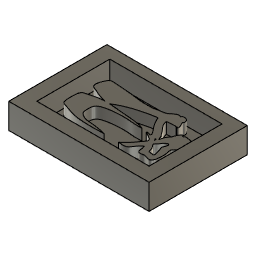
Pointe_Shoe (Autodesk Fusion 360 design; units mm, degrees)
Autodesk Fusion 360 part; units mm, degrees
sketch "Sketch1" plane through (0, 0, 0) normal (0, 0, 1) x (1, 0, 0)
  spline S0 degree 5 poles (-11.1843, -2.2894) (-11.167, -2.3096) (-11.1327, -2.3492) (-11.0825, -2.4064) (-11.0179, -2.4782) (-10.9409, -2.5607) (-10.8672, -2.6362) (-10.7955, -2.7054) (-10.7238, -2.7696) (-10.6489, -2.8307) (-10.5674, -2.891) (-10.4761, -2.9527) (-10.3728, -3.0176) (-10.2574, -3.0865) (-10.1318, -3.1589) (-9.9991, -3.2339) (-9.8634, -3.3097) (-9.7286, -3.3844) (-9.5981, -3.4561) (-9.4738, -3.5232) (-9.3565, -3.5843) (-9.2459, -3.6385) (-9.1414, -3.6849) (-9.0421, -3.7231) (-8.9473, -3.7527) (-8.8567, -3.7736) (-8.7873, -3.7834) (-8.7369, -3.7869) (-8.7041, -3.7874) (-8.6879, -3.7873) knots 0 0 0 0 0 0 0.04 0.08 0.12 0.16 0.2 0.24 0.28 0.32 0.36 0.4 0.44 0.48 0.52 0.56 0.6 0.64 0.68 0.72 0.76 0.8 0.84 0.88 0.92 0.96 1 1 1 1 1 1
  spline S1 degree 5 poles (4.0148, 3.4427) (3.8783, 3.4353) (3.6103, 3.4218) (3.2238, 3.4053) (2.7393, 3.3909) (2.1844, 3.3854) (1.6785, 3.3922) (1.218, 3.4101) (0.7966, 3.438) (0.405, 3.4734) (0.0299, 3.5135) (-0.3435, 3.5544) (-0.7292, 3.5927) (-1.138, 3.6252) (-1.5741, 3.6497) (-2.0345, 3.6652) (-2.512, 3.6716) (-2.9969, 3.6695) (-3.4802, 3.6596) (-3.9557, 3.6428) (-4.4224, 3.6197) (-4.8836, 3.5905) (-5.3447, 3.5552) (-5.8119, 3.5134) (-6.2904, 3.4642) (-6.7826, 3.4063) (-7.2875, 3.3381) (-7.8013, 3.2575) (-8.3174, 3.1622) (-8.8273, 3.0498) (-9.3207, 2.9176) (-9.7857, 2.763) (-10.21, 2.5834) (-10.5824, 2.3753) (-10.8943, 2.1343) (-11.1409, 1.8548) (-11.3232, 1.5288) (-11.4473, 1.1483) (-11.522, 0.7091) (-11.5571, 0.2147) (-11.5606, -0.3207) (-11.537, -0.8664) (-11.4865, -1.3808) (-11.4055, -1.8231) (-11.31, -2.0996) (-11.2166, -2.2572) (-11.1425, -2.3444) (-11.1014, -2.3849) (-11.0994, -2.3868) knots 0 0 0 0 0 0 0.014286 0.028571 0.042857 0.057143 0.071429 0.085714 0.1 0.114286 0.128571 0.142857 0.157143 0.171429 0.185714 0.2 0.214286 0.228571 0.242857 0.257143 0.271429 0.285714 0.3 0.314286 0.328571 0.342857 0.357143 0.371429 0.385714 0.4 0.414286 0.428571 0.442857 0.457143 0.471429 0.485714 0.5 0.514286 0.528571 0.542857 0.557143 0.571429 0.585714 0.6 0.614286 0.615002 0.615002 0.615002 0.615002 0.615002 0.615002
  line L0 (-12.4584, -1.0588) -> (-9.7404, -3.7149)
  spline S2 degree 5 poles (-8.6879, -3.7873) (-8.6225, -3.8062) (-8.4825, -3.8421) (-8.2453, -3.8901) (-7.8792, -3.9433) (-7.3672, -3.9951) (-6.8379, -4.0368) (-6.3286, -4.0733) (-5.87, -4.1091) (-5.4766, -4.1473) (-5.1428, -4.1887) (-4.851, -4.2334) (-4.5778, -4.2808) (-4.301, -4.3301) (-4.0067, -4.3817) (-3.6897, -4.4364) (-3.3499, -4.4957) (-2.9908, -4.5607) (-2.6162, -4.6327) (-2.2288, -4.7122) (-1.8301, -4.7996) (-1.503, -4.8758) (-1.2532, -4.9365) (-1.0847, -4.9786) (-1, -5) knots 0 0 0 0 0 0 0.05 0.1 0.15 0.2 0.25 0.3 0.35 0.4 0.45 0.5 0.55 0.6 0.65 0.7 0.75 0.8 0.85 0.9 0.95 1 1 1 1 1 1
  line L1 (-9.2399, -3.6277) -> (-8.1358, -3.9468)
  spline S3 degree 5 poles (9.6142, 10.026) (9.6212, 10.039) (9.6388, 10.0609) (9.6761, 10.0818) (9.7474, 10.0856) (9.8704, 10.0531) (10.0203, 9.9927) (10.1831, 9.923) (10.3362, 9.8739) (10.4544, 9.8782) (10.5157, 9.9641) (10.5061, 10.1473) (10.4263, 10.4231) (10.2881, 10.7708) (10.1115, 11.1587) (9.9211, 11.5502) (9.7427, 11.9083) (9.5999, 12.2013) (9.5109, 12.4077) (9.4852, 12.5219) (9.5196, 12.5594) (9.596, 12.5616) (9.6883, 12.5778) (9.7702, 12.6495) (9.8232, 12.7907) (9.8366, 12.9926) (9.8066, 13.2316) (9.7349, 13.4774) (9.6278, 13.7) (9.4957, 13.8772) (9.3512, 14.0031) (9.2077, 14.0835) (9.076, 14.1314) (8.9623, 14.1621) (8.8658, 14.1892) (8.7751, 14.2189) (8.673, 14.2508) (8.5433, 14.2803) (8.3765, 14.3002) (8.1778, 14.3029) (7.9662, 14.282) (7.7663, 14.2336) (7.6026, 14.1578) (7.4921, 14.06) (7.4383, 13.9526) (7.4236, 13.8563) (7.4193, 13.7932) (7.3957, 13.779) (7.3349, 13.8141) (7.2335, 13.883) (7.0966, 13.9633) (6.9346, 14.0313) (6.7579, 14.071) (6.5743, 14.0766) (6.3902, 14.0492) (6.2103, 13.9947) (6.0374, 13.9214) (5.8732, 13.8375) (5.7178, 13.7485) (5.5707, 13.6572) (5.4304, 13.5647) (5.2956, 13.4708) (5.1651, 13.3751) (5.0383, 13.2773) (4.9157, 13.1779) (4.7981, 13.0778) (4.6859, 12.9784) (4.5792, 12.8811) (4.4765, 12.7872) (4.375, 12.6976) (4.2709, 12.6132) (4.1603, 12.5345) (4.0392, 12.4619) (3.9047, 12.3958) (3.7548, 12.3363) (3.5884, 12.2835) (3.4417, 12.2467) (3.3239, 12.2222) (3.2419, 12.2072) (3.2, 12.2) knots 0 0 0 0 0 0 0.01333333 0.02666667 0.04 0.05333333 0.06666667 0.08 0.09333333 0.10666667 0.12 0.13333333 0.14666667 0.16 0.17333333 0.18666667 0.2 0.21333333 0.22666667 0.24 0.25333333 0.26666667 0.28 0.29333333 0.30666667 0.32 0.33333333 0.34666667 0.36 0.37333333 0.38666667 0.4 0.41333333 0.42666667 0.44 0.45333333 0.46666667 0.48 0.49333333 0.50666667 0.52 0.53333333 0.54666667 0.56 0.57333333 0.58666667 0.6 0.61333333 0.62666667 0.64 0.65333333 0.66666667 0.68 0.69333333 0.70666667 0.72 0.73333333 0.74666667 0.76 0.77333333 0.78666667 0.8 0.81333333 0.82666667 0.84 0.85333333 0.86666667 0.88 0.89333333 0.90666667 0.92 0.93333333 0.94666667 0.96 0.97333333 0.98666667 1 1 1 1 1 1
  spline S4 degree 5 poles (2, 12) (2.048, 12.008) (2.144, 12.024) (2.288, 12.048) (2.48, 12.08) (2.72, 12.12) (2.912, 12.152) (3.056, 12.176) (3.152, 12.192) (3.2, 12.2) knots 0 0 0 0 0 0 0.2 0.4 0.6 0.8 1 1 1 1 1 1
  spline S5 degree 5 poles (2, 12) (1.9505, 11.9948) (1.8529, 11.984) (1.7107, 11.9662) (1.5296, 11.9392) (1.3172, 11.9004) (1.118, 11.8567) (0.9303, 11.8092) (0.7508, 11.7593) (0.5745, 11.7095) (0.3951, 11.6629) (0.2065, 11.6225) (0.0045, 11.5906) (-0.2127, 11.5683) (-0.4425, 11.5551) (-0.6794, 11.549) (-0.9162, 11.5474) (-1.1452, 11.5472) (-1.3596, 11.5458) (-1.5546, 11.5413) (-1.7278, 11.5326) (-1.8481, 11.5219) (-1.9281, 11.5118) (-1.9768, 11.5041) (-2, 11.5) knots 0 0 0 0 0 0 0.05 0.1 0.15 0.2 0.25 0.3 0.35 0.4 0.45 0.5 0.55 0.6 0.65 0.7 0.75 0.8 0.85 0.9 0.95 1 1 1 1 1 1
  spline S6 degree 5 poles (-3.9672, 11.5464) (-4.025, 11.5517) (-4.1405, 11.5622) (-4.3137, 11.5779) (-4.5447, 11.599) (-4.8335, 11.6253) (-5.0645, 11.6463) (-5.2378, 11.662) (-5.3533, 11.6726) (-5.411, 11.6778) knots 0 0 0 0 0 0 0.2 0.4 0.6 0.8 1 1 1 1 1 1
  spline S7 degree 5 poles (-2, 11.5) (-2.1116, 11.5015) (-2.329, 11.5045) (-2.6376, 11.5094) (-3.0142, 11.5163) (-3.429, 11.5261) (-3.7945, 11.5378) (-4.1243, 11.5528) (-4.4418, 11.5739) (-4.7789, 11.6044) (-5.1685, 11.6476) (-5.6391, 11.7054) (-6.2075, 11.7775) (-6.8769, 11.8614) (-7.64, 11.9528) (-8.4809, 12.0469) (-9.3773, 12.1388) (-10.3028, 12.224) (-11.229, 12.2999) (-12.1273, 12.3657) (-12.9715, 12.4238) (-13.7395, 12.4772) (-14.4143, 12.5278) (-14.9866, 12.5734) (-15.4556, 12.6057) (-15.8312, 12.6081) (-16.1363, 12.5523) (-16.4047, 12.4001) (-16.6687, 12.1177) (-16.9492, 11.6855) (-17.242, 11.1144) (-17.518, 10.4443) (-17.7367, 9.7313) (-17.8546, 9.038) (-17.837, 8.4217) (-17.6665, 7.9249) (-17.3563, 7.5626) (-16.9522, 7.3178) (-16.5127, 7.1553) (-16.0928, 7.0332) (-15.7276, 6.9134) (-15.4118, 6.7751) (-15.1095, 6.6135) (-14.7757, 6.4337) (-14.3731, 6.2459) (-13.8942, 6.0591) (-13.3587, 5.8807) (-12.8024, 5.7165) (-12.2684, 5.5708) (-11.7983, 5.4466) (-11.4216, 5.346) (-11.206, 5.2849) (-11.0947, 5.2502) (-11.0428, 5.232) (-11.0225, 5.2241) knots 0 0 0 0 0 0 0.02 0.04 0.06 0.08 0.1 0.12 0.14 0.16 0.18 0.2 0.22 0.24 0.26 0.28 0.3 0.32 0.34 0.36 0.38 0.4 0.42 0.44 0.46 0.48 0.5 0.52 0.54 0.56 0.58 0.6 0.62 0.64 0.66 0.68 0.7 0.72 0.74 0.76 0.78 0.8 0.82 0.84 0.86 0.88 0.9 0.92 0.94 0.96 0.98 1 1 1 1 1 1
  spline S8 degree 5 poles (4.0148, 3.4427) (3.8887, 3.4949) (3.6281, 3.596) (3.2125, 3.7383) (2.609, 3.9092) (1.7731, 4.092) (0.8587, 4.2454) (-0.1284, 4.3727) (-1.1777, 4.479) (-2.2738, 4.5724) (-3.3981, 4.6617) (-4.5314, 4.7545) (-5.656, 4.8558) (-6.7583, 4.9655) (-7.6991, 5.0635) (-8.4088, 5.1313) (-8.9025, 5.1705) (-9.1876, 5.1893) (-9.2671, 5.1943) knots 0 0 0 0 0 0 0.02 0.04 0.06 0.08 0.1 0.12 0.14 0.16 0.18 0.2 0.22 0.24 0.26 0.267756 0.267756 0.267756 0.267756 0.267756 0.267756
  line L2 (-7.9272, 5.1108) -> (-10.607, 5.2777)
  spline S9 degree 5 poles (-11.0225, 5.2241) (-11.1998, 5.2175) (-11.5778, 5.1974) (-12.1554, 5.1467) (-12.9304, 5.0358) (-13.8902, 4.8332) (-14.8317, 4.5921) (-15.6961, 4.3582) (-16.4481, 4.1622) (-17.0602, 4.0074) (-17.5215, 3.8527) (-17.8464, 3.5928) (-18.063, 3.1132) (-18.2006, 2.3488) (-18.276, 1.3464) (-18.2953, 0.2279) (-18.2564, -0.8529) (-18.1506, -1.7534) (-17.9656, -2.3797) (-17.6869, -2.7412) (-17.3014, -2.936) (-16.8022, -3.0842) (-16.194, -3.2658) (-15.4925, -3.501) (-14.7183, -3.7779) (-13.8925, -4.065) (-13.0313, -4.3318) (-12.1419, -4.5616) (-11.2253, -4.7474) (-10.2782, -4.8895) (-9.2946, -4.9925) (-8.2679, -5.063) (-7.1931, -5.1062) (-6.0667, -5.1257) (-4.8865, -5.1242) (-3.6513, -5.103) (-2.6186, -5.0711) (-1.819, -5.0388) (-1.2749, -5.0135) (-1, -5) knots 0.302378 0.302378 0.302378 0.302378 0.302378 0.302378 0.32 0.34 0.36 0.38 0.4 0.42 0.44 0.46 0.48 0.5 0.52 0.54 0.56 0.58 0.6 0.62 0.64 0.66 0.68 0.7 0.72 0.74 0.76 0.78 0.8 0.82 0.84 0.86 0.88 0.9 0.92 0.94 0.96 0.98 1 1 1 1 1 1
  line L3 (-8.0902, 5.3338) -> (-13.9548, 5.1144)
  spline S10 degree 5 poles (6, 3) (6.1626, 2.9146) (6.4768, 2.7481) (6.9154, 2.5109) (7.4345, 2.2202) (7.9733, 1.8987) (8.402, 1.6171) (8.7212, 1.3715) (8.9327, 1.1545) (9.0401, 0.9549) (9.0495, 0.7564) (8.9696, 0.5377) (8.8115, 0.2784) (8.5885, -0.0363) (8.3157, -0.41) (8.0099, -0.831) (7.688, -1.2777) (7.3658, -1.7242) (7.0565, -2.1441) (6.7694, -2.5169) (6.5089, -2.8312) (6.2721, -3.0922) (6.0509, -3.3176) (5.8351, -3.5296) (5.6157, -3.7489) (5.3871, -3.9868) (5.1508, -4.2387) (4.9136, -4.4882) (4.6843, -4.7133) (4.4724, -4.8915) (4.2847, -5.0059) (4.1566, -5.0404) (4.0733, -5.0331) (4.0235, -5.0135) (4, -5) knots 0 0 0 0 0 0 0.033333 0.066667 0.1 0.133333 0.166667 0.2 0.233333 0.266667 0.3 0.333333 0.366667 0.4 0.433333 0.466667 0.5 0.533333 0.566667 0.6 0.633333 0.666667 0.7 0.733333 0.766667 0.8 0.833333 0.866667 0.9 0.933333 0.966667 1 1 1 1 1 1
  spline S11 degree 5 poles (4, -5) (4.139, -5.0271) (4.4102, -5.0769) (4.7968, -5.1386) (5.272, -5.1946) (5.798, -5.2201) (6.2563, -5.2007) (6.6483, -5.1361) (6.978, -5.0267) (7.2527, -4.8739) (7.4841, -4.6807) (7.6865, -4.4515) (7.8744, -4.1919) (8.0607, -3.9092) (8.2538, -3.6117) (8.4567, -3.3092) (8.6688, -3.0113) (8.8874, -2.7274) (9.1089, -2.4653) (9.3301, -2.2305) (9.5496, -2.0257) (9.723, -1.8869) (9.8518, -1.7968) (9.9371, -1.743) (9.9795, -1.7176) knots 0 0 0 0 0 0 0.05 0.1 0.15 0.2 0.25 0.3 0.35 0.4 0.45 0.5 0.55 0.6 0.65 0.7 0.75 0.8 0.85 0.9 0.95 1 1 1 1 1 1
  spline S12 degree 5 poles (9.9795, -1.7176) (10.007, -1.7591) (10.0593, -1.8449) (10.1302, -1.9818) (10.2093, -2.1805) (10.2836, -2.4553) (10.3358, -2.7536) (10.3713, -3.0703) (10.399, -3.3962) (10.4323, -3.718) (10.4889, -4.0175) (10.5867, -4.2761) (10.7397, -4.4772) (10.9544, -4.6101) (11.2261, -4.6727) (11.5348, -4.6753) (11.8525, -4.6359) (12.1494, -4.5765) (12.4017, -4.5184) (12.5975, -4.4787) (12.7461, -4.4649) (12.8756, -4.4749) (13.0176, -4.5023) (13.1945, -4.5414) (13.4082, -4.5905) (13.6485, -4.6499) (13.8992, -4.7195) (14.1443, -4.7974) (14.3753, -4.8773) (14.5923, -4.9485) (14.7994, -4.998) (15.0021, -5.012) (15.2039, -4.9775) (15.4032, -4.8836) (15.5949, -4.7227) (15.7723, -4.4905) (15.9284, -4.1875) (16.0579, -3.819) (16.1587, -3.3962) (16.2311, -2.9342) (16.2775, -2.4506) (16.3013, -1.964) (16.3068, -1.4918) (16.2982, -1.0495) (16.2791, -0.648) (16.2518, -0.2932) (16.2169, 0.0171) (16.1733, 0.2915) (16.1205, 0.5417) (16.0594, 0.7799) (15.9944, 1.0157) (15.9348, 1.2533) (15.8957, 1.4886) (15.8941, 1.7136) (15.944, 1.9204) (16.0533, 2.1048) (16.2178, 2.2714) (16.4225, 2.433) (16.6455, 2.6061) (16.8629, 2.8077) (17.0521, 3.051) (17.1965, 3.3418) (17.2881, 3.676) (17.3263, 4.0427) (17.3163, 4.427) (17.2675, 4.8126) (17.193, 5.1843) (17.1076, 5.5308) (17.0268, 5.8479) (16.9652, 6.1388) (16.9341, 6.4109) (16.9396, 6.6728) (16.9799, 6.9313) (17.0439, 7.189) (17.1076, 7.4404) (17.1394, 7.6743) (17.1081, 7.8784) (16.9897, 8.0428) (16.7757, 8.1648) (16.4779, 8.2513) (16.1214, 8.3138) (15.7388, 8.3653) (15.3647, 8.4156) (15.0294, 8.4679) (14.7536, 8.5145) (14.5417, 8.5325) (14.3854, 8.4955) (14.27, 8.3901) (14.1788, 8.229) (14.0986, 8.0682) (14.0201, 7.9758) (13.9378, 8.0005) (13.8508, 8.1322) (13.7599, 8.3177) (13.6644, 8.489) (13.5584, 8.5919) (13.4318, 8.5991) (13.2768, 8.5023) (13.095, 8.3094) (12.8978, 8.0404) (12.7013, 7.7226) (12.5229, 7.3861) (12.3767, 7.0599) (12.2701, 6.767) (12.1992, 6.5201) (12.1472, 6.3185) (12.092, 6.1524) (12.0125, 6.005) (11.8946, 5.8557) (11.7381, 5.6832) (11.5528, 5.4682) (11.3546, 5.1966) (11.1613, 4.863) (10.9895, 4.4738) (10.8497, 4.0497) (10.743, 3.6303) (10.6626, 3.2653) (10.5976, 3.0042) (10.5356, 2.8859) (10.4661, 2.9299) (10.3835, 3.1238) (10.289, 3.4209) (10.1873, 3.7583) (10.0847, 4.0718) (9.9859, 4.3119) (9.8927, 4.4585) (9.8003, 4.5387) (9.7017, 4.6029) (9.5911, 4.6998) (9.4688, 4.8471) (9.3399, 5.0359) (9.2108, 5.2442) (9.0872, 5.4472) (8.9707, 5.6301) (8.8586, 5.7918) (8.7459, 5.9382) (8.627, 6.0792) (8.4975, 6.2238) (8.3551, 6.3771) (8.1994, 6.542) (8.0316, 6.7198) (7.8541, 6.9107) (7.6704, 7.1148) (7.4844, 7.332) (7.3006, 7.5622) (7.1234, 7.8053) (6.9569, 8.061) (6.8042, 8.3293) (6.6678, 8.61) (6.5492, 8.903) (6.4492, 9.2082) (6.3846, 9.4622) (6.3448, 9.6582) (6.3221, 9.7914) (6.3117, 9.8585) knots 0 0 0 0 0 0 0.00666667 0.01333333 0.02 0.02666667 0.03333333 0.04 0.04666667 0.05333333 0.06 0.06666667 0.07333333 0.08 0.08666667 0.09333333 0.1 0.10666667 0.11333333 0.12 0.12666667 0.13333333 0.14 0.14666667 0.15333333 0.16 0.16666667 0.17333333 0.18 0.18666667 0.19333333 0.2 0.20666667 0.21333333 0.22 0.22666667 0.23333333 0.24 0.24666667 0.25333333 0.26 0.26666667 0.27333333 0.28 0.28666667 0.29333333 0.3 0.30666667 0.31333333 0.32 0.32666667 0.33333333 0.34 0.34666667 0.35333333 0.36 0.36666667 0.37333333 0.38 0.38666667 0.39333333 0.4 0.40666667 0.41333333 0.42 0.42666667 0.43333333 0.44 0.44666667 0.45333333 0.46 0.46666667 0.47333333 0.48 0.48666667 0.49333333 0.5 0.50666667 0.51333333 0.52 0.52666667 0.53333333 0.54 0.54666667 0.55333333 0.56 0.56666667 0.57333333 0.58 0.58666667 0.59333333 0.6 0.60666667 0.61333333 0.62 0.62666667 0.63333333 0.64 0.64666667 0.65333333 0.66 0.66666667 0.67333333 0.68 0.68666667 0.69333333 0.7 0.70666667 0.71333333 0.72 0.72666667 0.73333333 0.74 0.74666667 0.75333333 0.76 0.76666667 0.77333333 0.78 0.78666667 0.79333333 0.8 0.80666667 0.81333333 0.82 0.82666667 0.83333333 0.84 0.84666667 0.85333333 0.86 0.86666667 0.87333333 0.88 0.88666667 0.89333333 0.9 0.90666667 0.91333333 0.92 0.92666667 0.93333333 0.94 0.94666667 0.95333333 0.96 0.96666667 0.97333333 0.98 0.98666667 0.99333333 1 1 1 1 1 1
  spline S13 degree 5 poles (3.647, 9.5084) (3.6997, 9.4048) (3.8036, 9.2012) (3.9549, 8.9067) (4.1475, 8.5361) (4.3731, 8.1092) (4.5851, 7.7174) (4.7864, 7.3576) (4.9821, 7.0242) (5.18, 6.7081) (5.3915, 6.3963) (5.6285, 6.0741) (5.9003, 5.7283) (6.2099, 5.3505) (6.5513, 4.9396) (6.9054, 4.5052) (7.2378, 4.0701) (7.509, 3.6639) (7.682, 3.3177) (7.7318, 3.0586) (7.6526, 2.9042) (7.4715, 2.8572) (7.2359, 2.9006) (6.9925, 3.0029) (6.7534, 3.104) (6.5085, 3.152) (6.3085, 3.1318) (6.1553, 3.08) (6.052, 3.0294) (6, 3) knots 0 0 0 0 0 0 0.04 0.08 0.12 0.16 0.2 0.24 0.28 0.32 0.36 0.4 0.44 0.48 0.52 0.56 0.6 0.64 0.68 0.72 0.76 0.8 0.84 0.88 0.92 0.96 1 1 1 1 1 1
  spline S14 degree 5 poles (12.5, -2.5) (12.5233, -2.5221) (12.5764, -2.5576) (12.6791, -2.5879) (12.8741, -2.6023) (13.2276, -2.6385) (13.6618, -2.7155) (14.1182, -2.8167) (14.4335, -2.7691) (14.5235, -2.469) (14.4332, -1.9661) (14.2519, -1.3631) (14.0732, -0.7831) (13.957, -0.3209) (13.8354, 0.0299) (13.6935, 0.3071) (13.5613, 0.5552) (13.482, 0.8198) (13.4934, 1.1344) (13.5993, 1.5074) (13.7634, 1.9199) (13.93, 2.3368) (14.0378, 2.7149) (14.0372, 3.0127) (13.9044, 3.1987) (13.6595, 3.261) (13.349, 3.2039) (13.0268, 3.0432) (12.7361, 2.8022) (12.4889, 2.5074) (12.2749, 2.1861) (12.0723, 1.8633) (11.8595, 1.5598) (11.6247, 1.2896) (11.3796, 1.0566) (11.1608, 0.8544) (11.012, 0.6697) (10.9709, 0.4852) (11.0531, 0.2823) (11.2398, 0.0446) (11.4913, -0.2398) (11.7586, -0.5755) (11.9959, -0.9563) (12.1719, -1.3635) (12.2836, -1.7613) (12.3497, -2.1081) (12.3924, -2.3162) (12.4366, -2.4249) (12.4767, -2.4779) (12.5, -2.5) knots 0 0 0 0 0 0 0.022222 0.044444 0.066667 0.088889 0.111111 0.133333 0.155556 0.177778 0.2 0.222222 0.244444 0.266667 0.288889 0.311111 0.333333 0.355556 0.377778 0.4 0.422222 0.444444 0.466667 0.488889 0.511111 0.533333 0.555556 0.577778 0.6 0.622222 0.644444 0.666667 0.688889 0.711111 0.733333 0.755556 0.777778 0.8 0.822222 0.844444 0.866667 0.888889 0.911111 0.933333 0.955556 0.977778 1 1 1 1 1 1
  spline S15 degree 5 poles (-9.2671, 5.1943) (-9.0708, 5.3122) (-8.6752, 5.5444) (-8.0731, 5.8813) (-7.253, 6.3078) (-6.1987, 6.8025) (-5.1159, 7.2582) (-4.0063, 7.6744) (-2.8735, 8.051) (-1.7233, 8.3885) (-0.5646, 8.6883) (0.5918, 8.9527) (1.6767, 9.1722) (2.5141, 9.3239) (3.1134, 9.4242) (3.4878, 9.4837) (3.647, 9.5084) knots 0 0 0 0 0 0 0.05 0.1 0.15 0.2 0.25 0.3 0.35 0.4 0.45 0.5 0.55 0.587521 0.587521 0.587521 0.587521 0.587521 0.587521
  line L4 (2.3392, 9.3051) -> (4.9547, 9.7118)
  spline S16 degree 5 poles (6.3117, 9.8585) (6.407, 9.8686) (6.6776, 9.8964) (7.1098, 9.9374) (7.6776, 9.9835) (8.3399, 10.0226) (8.9853, 10.0411) (9.4334, 10.0366) (9.7314, 10.0225) (9.9133, 10.0083) (10, 10) knots 0.72327 0.72327 0.72327 0.72327 0.72327 0.72327 0.75 0.8 0.85 0.9 0.95 1 1 1 1 1 1
  line L5 (5.8982, 9.8149) -> (6.7253, 9.9021)
  line L6 (7.9699, 2.6099) -> (6.0301, 3.3901)
  line L7 (14.2611, -1.4231) -> (13.7389, 0.4231)
  line L8 (13.4227, -2.7289) -> (14.6526, -2.8257)
  line L9 (14.2611, -1.4231) -> (14.5, -2.8)
  line L10 (10, 2.5) -> (9.6005, 2.5993)
  line L11 (9.6005, 2.5993) -> (10, 2)
  line L12 (10, 2) -> (10, 2.5)
  point P0 (-0.1076, 4.3633)
  point P1 (-7.056, 4.9968)
  point P2 (-13.056, 4.9968)
  point P3 (-17.056, 3.9968)
  point P4 (-18.056, 2.9968)
  point P5 (-18.056, -2.0032)
  point P6 (-17.056, -3.0032)
  point P7 (-14.056, -4.0032)
  point P8 (-9.056, -5.0032)
  point P9 (0.7673, 3.4427)
  point P10 (-1.0205, 3.6145)
  point P11 (-3.5165, 3.6568)
  point P12 (-6.0548, 3.4876)
  point P13 (-9, 3)
  point P14 (-11, 2)
  point P15 (-11.5545, 0)
  point P16 (-11.1843, -2.2894)
  point P17 (-6, -4.1)
  point P18 (-4.4895, -4.2966)
  point P19 (-3.0511, -4.5505)
  point P20 (-10.8, -2.7)
  point P21 (-10.4, -3)
  point P22 (-9.7, -3.4)
  point P23 (-9.1, -3.7)
  point P24 (-3, 8)
  point P25 (8, 10)
  point P26 (10.5, 10)
  point P27 (9.5, 12.5)
  point P28 (9.7, 12.6)
  point P29 (9.6142, 13.701)
  point P30 (8.9417, 14.1681)
  point P31 (8.4633, 14.2877)
  point P32 (7.5, 14.05)
  point P33 (7.4041, 13.7923)
  point P34 (7, 14)
  point P35 (6, 13.9)
  point P36 (5.2, 13.4)
  point P37 (4.6, 12.9)
  point P38 (4.1, 12.5)
  point P39 (0.9, 11.8)
  point P40 (-0.0122, 11.5913)
  point P41 (-1.2257, 11.5464)
  point P42 (-11.2999, 12.3035)
  point P43 (-15.7, 12.6)
  point P44 (-16.8, 11.9)
  point P45 (-17.7, 8.1)
  point P46 (-16, 7)
  point P47 (-14.6566, 6.3821)
  point P48 (-12, 5.5)
  point P49 (9, 1)
  point P50 (8.6094, -0.0043)
  point P51 (6.6911, -2.6076)
  point P52 (5.595, -3.7723)
  point P53 (4.5331, -4.8342)
  point P54 (7, -5)
  point P55 (8, -4)
  point P56 (9.0204, -2.5734)
  point P57 (10.3906, -3.2927)
  point P58 (10.9729, -4.5944)
  point P59 (12.5, -4.5)
  point P60 (13, -4.5)
  point P61 (13.999, -4.7524)
  point P62 (15, -5)
  point P63 (15.9154, -4.1861)
  point P64 (16.2668, -0.5069)
  point P65 (16, 1)
  point P66 (16, 2)
  point P67 (17, 3)
  point P68 (17.1414, 5.3901)
  point P69 (17, 7)
  point P70 (17, 8)
  point P71 (15.0046, 8.4726)
  point P72 (14.269, 8.3675)
  point P73 (14, 8)
  point P74 (13.7086, 8.4025)
  point P75 (13.3583, 8.5427)
  point P76 (12.3074, 6.8613)
  point P77 (12, 6)
  point P78 (10.9763, 4.4093)
  point P79 (10.4859, 2.9381)
  point P80 (9.9795, 4.3042)
  point P81 (9.6756, 4.6297)
  point P82 (9.1529, 5.3391)
  point P83 (8.6675, 6.0298)
  point P84 (8.0141, 6.7392)
  point P85 (7, 8)
  point P86 (5, 7)
  point P87 (6.5, 5)
  point P88 (7.6836, 3.0081)
  point P89 (7, 3)
  point P90 (14.0376, -2.7773)
  point P91 (14, -0.5)
  point P92 (13.5, 1)
  point P93 (14, 3)
  point P94 (13, 3)
  point P95 (11.7119, 1.3968)
  point P96 (11, 0.5)
  point P97 (12, -1)
  constraint coincident P16 S0.start
  constraint coincident S0.end S2.start
  constraint coincident S0 S1.end
  constraint midpoint S1.end L0
  constraint midpoint S0.end L1
  constraint coincident S3.start S16
  constraint midpoint S8.end L2
  constraint midpoint S7.end L3
  constraint coincident S13.start S15.end
  constraint midpoint S13.start L4
  constraint midpoint S12.end L5
  constraint midpoint P89 L6
  constraint midpoint P91 L7
  constraint midpoint P90 L8
  constraint coincident L7.start L9.start
extrude "Extrude1" add sketch "Sketch1" along normal blind 2 contours S0 S1 S2 S8 L2 S9 L3 | L2 L3 S15 | S3 S4 S5 S7 L3 S10 S11 S12 S13 S15 S16 L5 makes body 1
sketch "Sketch2" plane through (0, 0, 2) normal (0, 0, 1) x (-1, 0, 0)
  spline S0 degree 5 poles (-12.5, 2.5) (-12.4767, 2.4779) (-12.4366, 2.4249) (-12.3924, 2.3162) (-12.3497, 2.1081) (-12.2836, 1.7613) (-12.1719, 1.3635) (-11.9959, 0.9563) (-11.7586, 0.5755) (-11.4913, 0.2398) (-11.2398, -0.0446) (-11.0531, -0.2823) (-10.9709, -0.4852) (-11.012, -0.6697) (-11.1608, -0.8544) (-11.3796, -1.0566) (-11.6247, -1.2896) (-11.8595, -1.5598) (-12.0723, -1.8633) (-12.2749, -2.1861) (-12.4889, -2.5074) (-12.7361, -2.8022) (-13.0268, -3.0432) (-13.349, -3.2039) (-13.6595, -3.261) (-13.9044, -3.1987) (-14.0372, -3.0127) (-14.0378, -2.7149) (-13.93, -2.3368) (-13.7634, -1.9199) (-13.5993, -1.5074) (-13.4934, -1.1344) (-13.482, -0.8198) (-13.5613, -0.5552) (-13.6935, -0.3071) (-13.8354, -0.0299) (-13.957, 0.3209) (-14.0732, 0.7831) (-14.2519, 1.3631) (-14.4332, 1.9661) (-14.5235, 2.469) (-14.4335, 2.7691) (-14.1182, 2.8167) (-13.6618, 2.7155) (-13.2276, 2.6385) (-12.8741, 2.6023) (-12.6791, 2.5879) (-12.5764, 2.5576) (-12.5233, 2.5221) (-12.5, 2.5) knots -1 -1 -1 -1 -1 -1 -0.977778 -0.955556 -0.933333 -0.911111 -0.888889 -0.866667 -0.844444 -0.822222 -0.8 -0.777778 -0.755556 -0.733333 -0.711111 -0.688889 -0.666667 -0.644444 -0.622222 -0.6 -0.577778 -0.555556 -0.533333 -0.511111 -0.488889 -0.466667 -0.444444 -0.422222 -0.4 -0.377778 -0.355556 -0.333333 -0.311111 -0.288889 -0.266667 -0.244444 -0.222222 -0.2 -0.177778 -0.155556 -0.133333 -0.111111 -0.088889 -0.066667 -0.044444 -0.022222 0 0 0 0 0 0
  line L0 (-10, -2.5) -> (-10, -2)
  line L1 (-10, -2) -> (-9.6005, -2.5993)
  line L2 (-9.6005, -2.5993) -> (-10, -2.5)
  spline S1 degree 5 poles (-4.0148, -3.4427) (-3.8887, -3.4949) (-3.6281, -3.596) (-3.2125, -3.7383) (-2.609, -3.9092) (-1.7731, -4.092) (-0.8587, -4.2454) (0.1284, -4.3727) (1.1777, -4.479) (2.2738, -4.5724) (3.3981, -4.6617) (4.5314, -4.7545) (5.656, -4.8558) (6.7583, -4.9655) (7.6991, -5.0635) (8.4088, -5.1313) (8.9025, -5.1705) (9.1876, -5.1893) (9.2671, -5.1943) knots 0 0 0 0 0 0 0.02 0.04 0.06 0.08 0.1 0.12 0.14 0.16 0.18 0.2 0.22 0.24 0.26 0.267756 0.267756 0.267756 0.267756 0.267756 0.267756
  spline S2 degree 5 poles (9.2671, -5.1943) (9.0708, -5.3122) (8.6752, -5.5444) (8.0731, -5.8813) (7.253, -6.3078) (6.1987, -6.8025) (5.1159, -7.2582) (4.0063, -7.6744) (2.8735, -8.051) (1.7233, -8.3885) (0.5646, -8.6883) (-0.5918, -8.9527) (-1.6767, -9.1722) (-2.5141, -9.3239) (-3.1134, -9.4242) (-3.4878, -9.4837) (-3.647, -9.5084) knots 0 0 0 0 0 0 0.05 0.1 0.15 0.2 0.25 0.3 0.35 0.4 0.45 0.5 0.55 0.587521 0.587521 0.587521 0.587521 0.587521 0.587521
  spline S3 degree 5 poles (-3.647, -9.5084) (-3.6997, -9.4048) (-3.8036, -9.2012) (-3.9549, -8.9067) (-4.1475, -8.5361) (-4.3731, -8.1092) (-4.5851, -7.7174) (-4.7864, -7.3576) (-4.9821, -7.0242) (-5.18, -6.7081) (-5.3915, -6.3963) (-5.6285, -6.0741) (-5.9003, -5.7283) (-6.2099, -5.3505) (-6.5513, -4.9396) (-6.9054, -4.5052) (-7.2378, -4.0701) (-7.509, -3.6639) (-7.682, -3.3177) (-7.7318, -3.0586) (-7.6526, -2.9042) (-7.4715, -2.8572) (-7.2359, -2.9006) (-6.9925, -3.0029) (-6.7534, -3.104) (-6.5085, -3.152) (-6.3085, -3.1318) (-6.1553, -3.08) (-6.052, -3.0294) (-6, -3) knots 0 0 0 0 0 0 0.04 0.08 0.12 0.16 0.2 0.24 0.28 0.32 0.36 0.4 0.44 0.48 0.52 0.56 0.6 0.64 0.68 0.72 0.76 0.8 0.84 0.88 0.92 0.96 1 1 1 1 1 1
  spline S4 degree 5 poles (-6, -3) (-6.1626, -2.9146) (-6.4768, -2.7481) (-6.9154, -2.5109) (-7.4345, -2.2202) (-7.9733, -1.8987) (-8.402, -1.6171) (-8.7212, -1.3715) (-8.9327, -1.1545) (-9.0401, -0.9549) (-9.0495, -0.7564) (-8.9696, -0.5377) (-8.8115, -0.2784) (-8.5885, 0.0363) (-8.3157, 0.41) (-8.0099, 0.831) (-7.688, 1.2777) (-7.3658, 1.7242) (-7.0565, 2.1441) (-6.7694, 2.5169) (-6.5089, 2.8312) (-6.2721, 3.0922) (-6.0509, 3.3176) (-5.8351, 3.5296) (-5.6157, 3.7489) (-5.3871, 3.9868) (-5.1508, 4.2387) (-4.9136, 4.4882) (-4.6843, 4.7133) (-4.4784, 4.8864) (-4.3329, 4.9765) (-4.2363, 5.0142) (-4.1784, 5.0262) (-4.1526, 5.029) knots 0 0 0 0 0 0 0.033333 0.066667 0.1 0.133333 0.166667 0.2 0.233333 0.266667 0.3 0.333333 0.366667 0.4 0.433333 0.466667 0.5 0.533333 0.566667 0.6 0.633333 0.666667 0.7 0.733333 0.766667 0.8 0.833333 0.866667 0.9 0.933333 0.961942 0.961942 0.961942 0.961942 0.961942 0.961942
  spline S5 degree 5 poles (-4.1526, 5.029) (-4.2584, 5.0486) (-4.4955, 5.0903) (-4.8494, 5.1447) (-5.2953, 5.1957) (-5.798, 5.2201) (-6.2563, 5.2007) (-6.6483, 5.1361) (-6.978, 5.0267) (-7.2527, 4.8739) (-7.4841, 4.6807) (-7.6865, 4.4515) (-7.8744, 4.1919) (-8.0607, 3.9092) (-8.2538, 3.6117) (-8.4567, 3.3092) (-8.6688, 3.0113) (-8.8874, 2.7274) (-9.1089, 2.4653) (-9.3301, 2.2305) (-9.5496, 2.0257) (-9.723, 1.8869) (-9.8518, 1.7968) (-9.9371, 1.743) (-9.9795, 1.7176) knots 0.011104 0.011104 0.011104 0.011104 0.011104 0.011104 0.05 0.1 0.15 0.2 0.25 0.3 0.35 0.4 0.45 0.5 0.55 0.6 0.65 0.7 0.75 0.8 0.85 0.9 0.95 1 1 1 1 1 1
  spline S6 degree 5 poles (-9.9795, 1.7176) (-10.007, 1.7591) (-10.0593, 1.8449) (-10.1302, 1.9818) (-10.2093, 2.1805) (-10.2836, 2.4553) (-10.3358, 2.7536) (-10.3713, 3.0703) (-10.399, 3.3962) (-10.4323, 3.718) (-10.4889, 4.0175) (-10.5867, 4.2761) (-10.7397, 4.4772) (-10.9544, 4.6101) (-11.2261, 4.6727) (-11.5348, 4.6753) (-11.8525, 4.6359) (-12.1494, 4.5765) (-12.4017, 4.5184) (-12.5975, 4.4787) (-12.7461, 4.4649) (-12.8756, 4.4749) (-13.0176, 4.5023) (-13.1945, 4.5414) (-13.4082, 4.5905) (-13.6485, 4.6499) (-13.8992, 4.7195) (-14.1443, 4.7974) (-14.3753, 4.8773) (-14.5923, 4.9485) (-14.7994, 4.998) (-15.0021, 5.012) (-15.2039, 4.9775) (-15.4032, 4.8836) (-15.5949, 4.7227) (-15.7723, 4.4905) (-15.9284, 4.1875) (-16.0579, 3.819) (-16.1587, 3.3962) (-16.2311, 2.9342) (-16.2775, 2.4506) (-16.3013, 1.964) (-16.3068, 1.4918) (-16.2982, 1.0495) (-16.2791, 0.648) (-16.2518, 0.2932) (-16.2169, -0.0171) (-16.1733, -0.2915) (-16.1205, -0.5417) (-16.0594, -0.7799) (-15.9944, -1.0157) (-15.9348, -1.2533) (-15.8957, -1.4886) (-15.8941, -1.7136) (-15.944, -1.9204) (-16.0533, -2.1048) (-16.2178, -2.2714) (-16.4225, -2.433) (-16.6455, -2.6061) (-16.8629, -2.8077) (-17.0521, -3.051) (-17.1965, -3.3418) (-17.2881, -3.676) (-17.3263, -4.0427) (-17.3163, -4.427) (-17.2675, -4.8126) (-17.193, -5.1843) (-17.1076, -5.5308) (-17.0268, -5.8479) (-16.9652, -6.1388) (-16.9341, -6.4109) (-16.9396, -6.6728) (-16.9799, -6.9313) (-17.0439, -7.189) (-17.1076, -7.4404) (-17.1394, -7.6743) (-17.1081, -7.8784) (-16.9897, -8.0428) (-16.7757, -8.1648) (-16.4779, -8.2513) (-16.1214, -8.3138) (-15.7388, -8.3653) (-15.3647, -8.4156) (-15.0294, -8.4679) (-14.7536, -8.5145) (-14.5417, -8.5325) (-14.3854, -8.4955) (-14.27, -8.3901) (-14.1788, -8.229) (-14.0986, -8.0682) (-14.0201, -7.9758) (-13.9378, -8.0005) (-13.8508, -8.1322) (-13.7599, -8.3177) (-13.6644, -8.489) (-13.5584, -8.5919) (-13.4318, -8.5991) (-13.2768, -8.5023) (-13.095, -8.3094) (-12.8978, -8.0404) (-12.7013, -7.7226) (-12.5229, -7.3861) (-12.3767, -7.0599) (-12.2701, -6.767) (-12.1992, -6.5201) (-12.1472, -6.3185) (-12.092, -6.1524) (-12.0125, -6.005) (-11.8946, -5.8557) (-11.7381, -5.6832) (-11.5528, -5.4682) (-11.3546, -5.1966) (-11.1613, -4.863) (-10.9895, -4.4738) (-10.8497, -4.0497) (-10.743, -3.6303) (-10.6626, -3.2653) (-10.5976, -3.0042) (-10.5356, -2.8859) (-10.4661, -2.9299) (-10.3835, -3.1238) (-10.289, -3.4209) (-10.1873, -3.7583) (-10.0847, -4.0718) (-9.9859, -4.3119) (-9.8927, -4.4585) (-9.8003, -4.5387) (-9.7017, -4.6029) (-9.5911, -4.6998) (-9.4688, -4.8471) (-9.3399, -5.0359) (-9.2108, -5.2442) (-9.0872, -5.4472) (-8.9707, -5.6301) (-8.8586, -5.7918) (-8.7459, -5.9382) (-8.627, -6.0792) (-8.4975, -6.2238) (-8.3551, -6.3771) (-8.1994, -6.542) (-8.0316, -6.7198) (-7.8541, -6.9107) (-7.6704, -7.1148) (-7.4844, -7.332) (-7.3006, -7.5622) (-7.1234, -7.8053) (-6.9569, -8.061) (-6.8042, -8.3293) (-6.6678, -8.61) (-6.5492, -8.903) (-6.4492, -9.2082) (-6.3846, -9.4622) (-6.3448, -9.6582) (-6.3221, -9.7914) (-6.3117, -9.8585) knots 0 0 0 0 0 0 0.00666667 0.01333333 0.02 0.02666667 0.03333333 0.04 0.04666667 0.05333333 0.06 0.06666667 0.07333333 0.08 0.08666667 0.09333333 0.1 0.10666667 0.11333333 0.12 0.12666667 0.13333333 0.14 0.14666667 0.15333333 0.16 0.16666667 0.17333333 0.18 0.18666667 0.19333333 0.2 0.20666667 0.21333333 0.22 0.22666667 0.23333333 0.24 0.24666667 0.25333333 0.26 0.26666667 0.27333333 0.28 0.28666667 0.29333333 0.3 0.30666667 0.31333333 0.32 0.32666667 0.33333333 0.34 0.34666667 0.35333333 0.36 0.36666667 0.37333333 0.38 0.38666667 0.39333333 0.4 0.40666667 0.41333333 0.42 0.42666667 0.43333333 0.44 0.44666667 0.45333333 0.46 0.46666667 0.47333333 0.48 0.48666667 0.49333333 0.5 0.50666667 0.51333333 0.52 0.52666667 0.53333333 0.54 0.54666667 0.55333333 0.56 0.56666667 0.57333333 0.58 0.58666667 0.59333333 0.6 0.60666667 0.61333333 0.62 0.62666667 0.63333333 0.64 0.64666667 0.65333333 0.66 0.66666667 0.67333333 0.68 0.68666667 0.69333333 0.7 0.70666667 0.71333333 0.72 0.72666667 0.73333333 0.74 0.74666667 0.75333333 0.76 0.76666667 0.77333333 0.78 0.78666667 0.79333333 0.8 0.80666667 0.81333333 0.82 0.82666667 0.83333333 0.84 0.84666667 0.85333333 0.86 0.86666667 0.87333333 0.88 0.88666667 0.89333333 0.9 0.90666667 0.91333333 0.92 0.92666667 0.93333333 0.94 0.94666667 0.95333333 0.96 0.96666667 0.97333333 0.98 0.98666667 0.99333333 1 1 1 1 1 1
  spline S7 degree 5 poles (-6.3117, -9.8585) (-6.407, -9.8686) (-6.6776, -9.8964) (-7.1098, -9.9374) (-7.6776, -9.9835) (-8.3399, -10.0226) (-8.8789, -10.0381) (-9.2459, -10.0376) (-9.4773, -10.0317) (-9.5965, -10.0268) (-9.6142, -10.026) knots 0.72327 0.72327 0.72327 0.72327 0.72327 0.72327 0.75 0.8 0.85 0.9 0.95 0.958807 0.958807 0.958807 0.958807 0.958807 0.958807
  spline S8 degree 5 poles (-9.6142, -10.026) (-9.6212, -10.039) (-9.6388, -10.0609) (-9.6761, -10.0818) (-9.7447, -10.0854) (-9.8383, -10.0616) (-9.9187, -10.0324) (-9.9741, -10.0105) (-10, -10) knots 0 0 0 0 0 0 0.013333 0.026667 0.04 0.051304 0.051304 0.051304 0.051304 0.051304 0.051304
  spline S9 degree 5 poles (-10, -10) (-10.0047, -9.9981) (-10.04, -9.9838) (-10.1077, -9.9559) (-10.209, -9.9147) (-10.3362, -9.8739) (-10.4544, -9.8782) (-10.5157, -9.9641) (-10.5061, -10.1473) (-10.4263, -10.4231) (-10.2881, -10.7708) (-10.1115, -11.1587) (-9.9211, -11.5502) (-9.7427, -11.9083) (-9.5999, -12.2013) (-9.5109, -12.4077) (-9.4852, -12.5219) (-9.5196, -12.5594) (-9.596, -12.5616) (-9.6883, -12.5778) (-9.7702, -12.6495) (-9.8232, -12.7907) (-9.8366, -12.9926) (-9.8066, -13.2316) (-9.7349, -13.4774) (-9.6278, -13.7) (-9.4957, -13.8772) (-9.3512, -14.0031) (-9.2077, -14.0835) (-9.076, -14.1314) (-8.9623, -14.1621) (-8.8658, -14.1892) (-8.7751, -14.2189) (-8.673, -14.2508) (-8.5433, -14.2803) (-8.3765, -14.3002) (-8.1778, -14.3029) (-7.9662, -14.282) (-7.7663, -14.2336) (-7.6026, -14.1578) (-7.4921, -14.06) (-7.4383, -13.9526) (-7.4236, -13.8563) (-7.4193, -13.7932) (-7.3957, -13.779) (-7.3349, -13.8141) (-7.2335, -13.883) (-7.0966, -13.9633) (-6.9346, -14.0313) (-6.7579, -14.071) (-6.5743, -14.0766) (-6.3902, -14.0492) (-6.2103, -13.9947) (-6.0374, -13.9214) (-5.8732, -13.8375) (-5.7178, -13.7485) (-5.5707, -13.6572) (-5.4304, -13.5647) (-5.2956, -13.4708) (-5.1651, -13.3751) (-5.0383, -13.2773) (-4.9157, -13.1779) (-4.7981, -13.0778) (-4.6859, -12.9784) (-4.5792, -12.8811) (-4.4765, -12.7872) (-4.375, -12.6976) (-4.2709, -12.6132) (-4.1603, -12.5345) (-4.0392, -12.4619) (-3.9047, -12.3958) (-3.7548, -12.3363) (-3.5884, -12.2835) (-3.4417, -12.2467) (-3.3239, -12.2222) (-3.2419, -12.2072) (-3.2, -12.2) knots 0.05130355 0.05130355 0.05130355 0.05130355 0.05130355 0.05130355 0.05333333 0.06666667 0.08 0.09333333 0.10666667 0.12 0.13333333 0.14666667 0.16 0.17333333 0.18666667 0.2 0.21333333 0.22666667 0.24 0.25333333 0.26666667 0.28 0.29333333 0.30666667 0.32 0.33333333 0.34666667 0.36 0.37333333 0.38666667 0.4 0.41333333 0.42666667 0.44 0.45333333 0.46666667 0.48 0.49333333 0.50666667 0.52 0.53333333 0.54666667 0.56 0.57333333 0.58666667 0.6 0.61333333 0.62666667 0.64 0.65333333 0.66666667 0.68 0.69333333 0.70666667 0.72 0.73333333 0.74666667 0.76 0.77333333 0.78666667 0.8 0.81333333 0.82666667 0.84 0.85333333 0.86666667 0.88 0.89333333 0.90666667 0.92 0.93333333 0.94666667 0.96 0.97333333 0.98666667 1 1 1 1 1 1
  line L3 (-3.2, -12.2) -> (-2, -12)
  spline S10 degree 5 poles (-2, -12) (-1.9505, -11.9948) (-1.8529, -11.984) (-1.7107, -11.9662) (-1.5296, -11.9392) (-1.3172, -11.9004) (-1.118, -11.8567) (-0.9303, -11.8092) (-0.7508, -11.7593) (-0.5745, -11.7095) (-0.3951, -11.6629) (-0.2065, -11.6225) (-0.0045, -11.5906) (0.2127, -11.5683) (0.4425, -11.5551) (0.6794, -11.549) (0.9162, -11.5474) (1.1452, -11.5472) (1.3596, -11.5458) (1.5546, -11.5413) (1.7278, -11.5326) (1.8481, -11.5219) (1.9281, -11.5118) (1.9768, -11.5041) (2, -11.5) knots 0 0 0 0 0 0 0.05 0.1 0.15 0.2 0.25 0.3 0.35 0.4 0.45 0.5 0.55 0.6 0.65 0.7 0.75 0.8 0.85 0.9 0.95 1 1 1 1 1 1
  spline S11 degree 5 poles (2, -11.5) (2.1116, -11.5015) (2.329, -11.5045) (2.6376, -11.5094) (3.0142, -11.5163) (3.429, -11.5261) (3.7945, -11.5378) (4.1243, -11.5528) (4.4418, -11.5739) (4.7789, -11.6044) (5.1685, -11.6476) (5.6391, -11.7054) (6.2075, -11.7775) (6.8769, -11.8614) (7.64, -11.9528) (8.4809, -12.0469) (9.3773, -12.1388) (10.3028, -12.224) (11.229, -12.2999) (12.1273, -12.3657) (12.9715, -12.4238) (13.7395, -12.4772) (14.4143, -12.5278) (14.9866, -12.5734) (15.4556, -12.6057) (15.8312, -12.6081) (16.1363, -12.5523) (16.4047, -12.4001) (16.6687, -12.1177) (16.9492, -11.6855) (17.242, -11.1144) (17.518, -10.4443) (17.7367, -9.7313) (17.8546, -9.038) (17.837, -8.4217) (17.6665, -7.9249) (17.3563, -7.5626) (16.9522, -7.3178) (16.5127, -7.1553) (16.0928, -7.0332) (15.7276, -6.9134) (15.4118, -6.7751) (15.1095, -6.6135) (14.7757, -6.4337) (14.3731, -6.2459) (13.8942, -6.0591) (13.3587, -5.8807) (12.8024, -5.7165) (12.2684, -5.5708) (11.7983, -5.4466) (11.4216, -5.346) (11.206, -5.2849) (11.0947, -5.2502) (11.0428, -5.232) (11.0225, -5.2241) knots 0 0 0 0 0 0 0.02 0.04 0.06 0.08 0.1 0.12 0.14 0.16 0.18 0.2 0.22 0.24 0.26 0.28 0.3 0.32 0.34 0.36 0.38 0.4 0.42 0.44 0.46 0.48 0.5 0.52 0.54 0.56 0.58 0.6 0.62 0.64 0.66 0.68 0.7 0.72 0.74 0.76 0.78 0.8 0.82 0.84 0.86 0.88 0.9 0.92 0.94 0.96 0.98 1 1 1 1 1 1
  spline S12 degree 5 poles (11.0225, -5.2241) (11.1998, -5.2175) (11.5778, -5.1974) (12.1554, -5.1467) (12.9304, -5.0358) (13.8902, -4.8332) (14.8317, -4.5921) (15.6961, -4.3582) (16.4481, -4.1622) (17.0602, -4.0074) (17.5215, -3.8527) (17.8464, -3.5928) (18.063, -3.1132) (18.2006, -2.3488) (18.276, -1.3464) (18.2953, -0.2279) (18.2564, 0.8529) (18.1506, 1.7534) (17.9656, 2.3797) (17.6869, 2.7412) (17.3014, 2.936) (16.8022, 3.0842) (16.194, 3.2658) (15.4925, 3.501) (14.7183, 3.7779) (13.8925, 4.065) (13.0313, 4.3318) (12.1419, 4.5616) (11.2253, 4.7474) (10.2782, 4.8895) (9.2946, 4.9925) (8.2679, 5.063) (7.1931, 5.1062) (6.0667, 5.1257) (4.8865, 5.1242) (3.6513, 5.103) (2.6186, 5.0711) (1.819, 5.0388) (1.2749, 5.0135) (1, 5) knots 0.302378 0.302378 0.302378 0.302378 0.302378 0.302378 0.32 0.34 0.36 0.38 0.4 0.42 0.44 0.46 0.48 0.5 0.52 0.54 0.56 0.58 0.6 0.62 0.64 0.66 0.68 0.7 0.72 0.74 0.76 0.78 0.8 0.82 0.84 0.86 0.88 0.9 0.92 0.94 0.96 0.98 1 1 1 1 1 1
  spline S13 degree 5 poles (1, 5) (1.0847, 4.9786) (1.2532, 4.9365) (1.503, 4.8758) (1.8301, 4.7996) (2.2288, 4.7122) (2.6162, 4.6327) (2.9908, 4.5607) (3.3499, 4.4957) (3.6897, 4.4364) (4.0067, 4.3817) (4.301, 4.3301) (4.5778, 4.2808) (4.851, 4.2334) (5.1428, 4.1887) (5.4766, 4.1473) (5.87, 4.1091) (6.3286, 4.0733) (6.8379, 4.0368) (7.3672, 3.9951) (7.8792, 3.9433) (8.2453, 3.8901) (8.4825, 3.8421) (8.6225, 3.8062) (8.6879, 3.7873) knots -1 -1 -1 -1 -1 -1 -0.95 -0.9 -0.85 -0.8 -0.75 -0.7 -0.65 -0.6 -0.55 -0.5 -0.45 -0.4 -0.35 -0.3 -0.25 -0.2 -0.15 -0.1 -0.05 0 0 0 0 0 0
  spline S14 degree 5 poles (8.6879, 3.7873) (8.7041, 3.7874) (8.7369, 3.7869) (8.7873, 3.7834) (8.8567, 3.7736) (8.9473, 3.7527) (9.0421, 3.7231) (9.1414, 3.6849) (9.2459, 3.6385) (9.3565, 3.5843) (9.4738, 3.5232) (9.5981, 3.4561) (9.7286, 3.3844) (9.8634, 3.3097) (9.9991, 3.2339) (10.1318, 3.1589) (10.2574, 3.0865) (10.3728, 3.0176) (10.4761, 2.9527) (10.5674, 2.891) (10.6489, 2.8307) (10.7238, 2.7696) (10.7955, 2.7054) (10.8672, 2.6362) (10.9409, 2.5608) (11.0024, 2.4948) (11.0502, 2.4421) (11.0829, 2.4055) (11.0994, 2.3868) knots -1 -1 -1 -1 -1 -1 -0.96 -0.92 -0.88 -0.84 -0.8 -0.76 -0.72 -0.68 -0.64 -0.6 -0.56 -0.52 -0.48 -0.44 -0.4 -0.36 -0.32 -0.28 -0.24 -0.2 -0.16 -0.12 -0.08 -0.040102 -0.040102 -0.040102 -0.040102 -0.040102 -0.040102
  spline S15 degree 5 poles (11.0994, 2.3868) (11.1014, 2.3849) (11.1195, 2.367) (11.137, 2.3484) (11.1539, 2.3289) (11.1702, 2.3084) (11.1843, 2.2894) knots -0.615002 -0.615002 -0.615002 -0.615002 -0.615002 -0.615002 -0.614286 -0.608391 -0.608391 -0.608391 -0.608391 -0.608391 -0.608391
  spline S16 degree 5 poles (11.1843, 2.2894) (11.2044, 2.2623) (11.2562, 2.185) (11.3303, 2.039) (11.4122, 1.7866) (11.4865, 1.3808) (11.537, 0.8664) (11.5606, 0.3207) (11.5571, -0.2147) (11.522, -0.7091) (11.4473, -1.1483) (11.3232, -1.5288) (11.1409, -1.8548) (10.8943, -2.1343) (10.5824, -2.3753) (10.21, -2.5834) (9.7857, -2.763) (9.3207, -2.9176) (8.8273, -3.0498) (8.3174, -3.1622) (7.8013, -3.2575) (7.2875, -3.3381) (6.7826, -3.4063) (6.2904, -3.4642) (5.8119, -3.5134) (5.3447, -3.5552) (4.8836, -3.5905) (4.4224, -3.6197) (3.9557, -3.6428) (3.4802, -3.6596) (2.9969, -3.6695) (2.512, -3.6716) (2.0345, -3.6652) (1.5741, -3.6497) (1.138, -3.6252) (0.7292, -3.5927) (0.3435, -3.5544) (-0.0299, -3.5135) (-0.405, -3.4734) (-0.7966, -3.438) (-1.218, -3.4101) (-1.6785, -3.3922) (-2.1844, -3.3854) (-2.7393, -3.3909) (-3.2238, -3.4053) (-3.6103, -3.4218) (-3.8783, -3.4353) (-4.0148, -3.4427) knots -0.608391 -0.608391 -0.608391 -0.608391 -0.608391 -0.608391 -0.6 -0.585714 -0.571429 -0.557143 -0.542857 -0.528571 -0.514286 -0.5 -0.485714 -0.471429 -0.457143 -0.442857 -0.428571 -0.414286 -0.4 -0.385714 -0.371429 -0.357143 -0.342857 -0.328571 -0.314286 -0.3 -0.285714 -0.271429 -0.257143 -0.242857 -0.228571 -0.214286 -0.2 -0.185714 -0.171429 -0.157143 -0.142857 -0.128571 -0.114286 -0.1 -0.085714 -0.071429 -0.057143 -0.042857 -0.028571 -0.014286 0 0 0 0 0 0
  line L4 (20, 10) -> (-20, 10)
  line L5 (-20, 10) -> (-20, -16)
  line L6 (-20, -16) -> (20, -16)
  line L7 (20, -16) -> (20, 10)
  line L8 (-25, 15) -> (25, 15)
  line L9 (25, 15) -> (25, -20)
  line L10 (25, -20) -> (-25, -20)
  line L11 (-25, -20) -> (-25, 15)
  constraint horizontal L4
  constraint vertical L5
  constraint horizontal L6
  constraint vertical L7
  constraint horizontal L8
  constraint vertical L9
  constraint horizontal L10
  constraint vertical L11
extrude "Extrude2" add sketch "Sketch2" along normal blind 30 separate body contours L8 L9 L10 L11 makes body 2
extrude "Extrude3" add 1 faces at (-6.4826, 10.2932, 2) along direction (0, 0, 1) blind 2 on bodies 1 bodies 1
sketch "Sketch3" plane through (0, 0, 0) normal (0, 0, 1) x (1, 0, 0)
  line L0 (-20, -10) -> (20, -10)
  line L1 (20, -10) -> (20, 16)
  line L2 (20, 16) -> (-20, 16)
  line L3 (-20, 16) -> (-20, -10)
  constraint horizontal L0
  constraint vertical L1
  constraint horizontal L2
  constraint vertical L3
extrude "Extrude4" cut sketch "Sketch3" along normal blind 2 bodies 1
sketch "Sketch4" plane through (0, 0, 0) normal (0, 0, 1) x (1, 0, 0)
  line L0 (-25, -15) -> (25, -15)
  line L1 (25, -15) -> (25, 20)
  line L2 (25, 20) -> (-25, 20)
  line L3 (-25, 20) -> (-25, -15)
  constraint horizontal L0
  constraint vertical L1
  constraint horizontal L2
  constraint vertical L3
extrude "Extrude5" add sketch "Sketch4" along normal blind 2 bodies 1 2
extrude "Extrude6" add 1 faces at (-6.4826, 10.2932, 4) along direction (0, 0, 1) blind 4 on bodies 1 bodies 1
extrude "Extrude7" cut 1 faces at (6.6667, -13.3333, 32) along direction (0, 0, -1) blind 10 on bodies 1 bodies 1
extrude "Extrude8" cut 1 faces at (6.6667, -13.3333, 22) along direction (0, 0, -1) blind 5 on bodies 1 bodies 1
extrude "Extrude9" cut 1 faces at (-6.4826, 10.2932, 8) along direction (0, 0, -1) blind 1 on bodies 1 bodies 1
extrude "Extrude10" add 1 faces at (-6.4826, 10.2932, 7) along direction (0, 0, -1) blind 5 on bodies 1 bodies 1
extrude "Extrude11" add 1 faces at (-6.4826, 10.2932, 7) along direction (0, 0, -1) blind 5 on bodies 1 bodies 1
extrude "Extrude12" cut 1 faces at (6.6667, -13.3333, 17) along direction (0, 0, -1) blind 6 on bodies 1 bodies 1
extrude "Extrude13" cut 1 faces at (-6.4826, 10.2932, 7) along direction (0, 0, -1) blind 1 on bodies 1 bodies 1
extrude "Extrude14" cut 1 faces at (6.6667, -13.3333, 11) along direction (0, 0, -1) blind 2 on bodies 1 bodies 1
